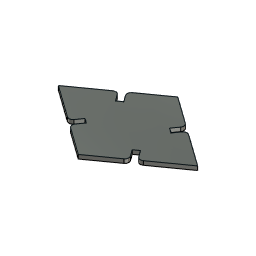
DukasPressFit v4 (Autodesk Fusion 360 design; units mm, degrees)
Autodesk Fusion 360 part; units mm, degrees
sketch "Sketch1" plane through (0, 0, 0) normal (0, 0, 1) x (1, 0, 0)
  line L0 (-17.4507, -12.5352) -> (-13.9632, -7.6528)
  line L1 (-13.9632, -7.6528) -> (-11.6848, -9.2803)
  line L2 (-11.6848, -9.2803) -> (-15.1722, -14.1627)
  line L3 (17.4507, -12.5352) -> (13.9632, -7.6528)
  line L4 (13.9632, -7.6528) -> (11.522, -9.3966)
  line L5 (11.522, -9.3966) -> (15.0095, -14.279)
  line L6 (11.522, 9.3966) -> (15.0095, 14.279)
  line L7 (13.9632, 7.6528) -> (11.522, 9.3966)
  line L8 (17.4507, 12.5352) -> (13.9632, 7.6528)
  line L9 (-11.522, 9.3966) -> (-15.0095, 14.279)
  line L10 (-13.9632, 7.6528) -> (-11.522, 9.3966)
  line L11 (-17.4507, 12.5352) -> (-13.9632, 7.6528)
  line L12 (-35, 0) -> (-17.4507, 12.5352)
  line L13 (-15.0095, 14.279) -> (0, 25)
  line L14 (0, 25) -> (15.0095, 14.279)
  line L15 (17.4507, 12.5352) -> (35, 0)
  line L16 (35, 0) -> (17.4507, -12.5352)
  line L17 (15.0095, -14.279) -> (0, -25)
  line L18 (-35, 0) -> (-17.4507, -12.5352)
  line L19 (-15.1722, -14.1627) -> (0, -25)
  dimension "d26" = 50
  constraint perpendicular L0 L1
  constraint perpendicular L9 L13
  constraint perpendicular L5 L17
  constraint perpendicular L0 L18
  constraint perpendicular L2 L19
  measures "d26" distance of L13.end L17.end
extrude "Extrude1" add sketch "Sketch1" along normal blind 2
fillet "Fillet1" radius 2 8 edges at (-15.0095, 14.279, 1) (-17.4507, 12.5352, 1) (-15.1722, -14.1627, 1) (-17.4507, -12.5352, 1) (15.0095, 14.279, 1) (17.4507, 12.5352, 1) (15.0095, -14.279, 1) (17.4507, -12.5352, 1)
sketch "Sketch2" plane through (0, 0, 2) normal (0, 0, 1) x (-1, 0, 0)
  arc A0 (-16.2882, 10.9078) -> (-19.0781, 11.3728) centre (-17.9157, 9.7453) ccw
  line L0 (-19.0781, 11.3728) -> (-35, 0)
  line L1 (-35, 0) -> (-19.0781, -11.3728)
  arc A1 (-19.0781, -11.3728) -> (-16.2882, -10.9078) centre (-17.9157, -9.7453) ccw
  line L2 (-16.2882, -10.9078) -> (-13.9632, -7.6528)
  line L3 (-13.9632, -7.6528) -> (-11.522, -9.3966)
  line L4 (-11.522, -9.3966) -> (-13.847, -12.6515)
  arc A2 (-13.847, -12.6515) -> (-13.382, -15.4414) centre (-12.2195, -13.814) ccw
  line L5 (-13.382, -15.4414) -> (0, -25)
  line L6 (0, -25) -> (13.382, -15.4414)
  arc A3 (13.382, -15.4414) -> (13.847, -12.6515) centre (12.2195, -13.814) ccw
  line L7 (13.847, -12.6515) -> (11.522, -9.3966)
  line L8 (11.522, -9.3966) -> (13.9632, -7.6528)
  line L9 (13.9632, -7.6528) -> (16.2882, -10.9078)
  arc A4 (16.2882, -10.9078) -> (19.0781, -11.3728) centre (17.9157, -9.7453) ccw
  line L10 (19.0781, -11.3728) -> (35, 0)
  line L11 (35, 0) -> (19.0781, 11.3728)
  arc A5 (19.0781, 11.3728) -> (16.2882, 10.9078) centre (17.9157, 9.7453) ccw
  line L12 (16.2882, 10.9078) -> (13.9632, 7.6528)
  line L13 (13.9632, 7.6528) -> (11.6848, 9.2803)
  line L14 (11.6848, 9.2803) -> (14.0097, 12.5352)
  arc A6 (14.0097, 12.5352) -> (13.5447, 15.3252) centre (12.3823, 13.6977) ccw
  line L15 (13.5447, 15.3252) -> (0, 25)
  line L16 (0, 25) -> (-13.382, 15.4414)
  arc A7 (-13.382, 15.4414) -> (-13.847, 12.6515) centre (-12.2195, 13.814) ccw
  line L17 (-13.847, 12.6515) -> (-11.522, 9.3966)
  line L18 (-11.522, 9.3966) -> (-13.9632, 7.6528)
  line L19 (-13.9632, 7.6528) -> (-16.2882, 10.9078)
equation "Kerf = 1 mm"
equation "thickness = 3.8 mm"
equation "long = 6.00 mm"
equation "d31 = ( thickness - Kerf )"
